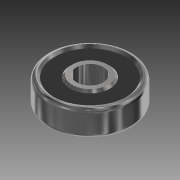
# Autodesk Inventor part: Roulement
Saved by Autodesk Inventor 2016 (Build 200138000, 138)
## iProperties
Created: 2015-04-27
Part Number: Roulement
Material: Générique
Document SubType Name: Modeling
Designer: Logan
Density: 1 g/cm^3
Appearance: Par défaut
Author: Logan
Autodesk Inventor part; units mm, degrees
ref_plane "YZ Plane" through (0, 0, 0) normal (1, 0, 0) x (0, 1, 0)
ref_plane "XZ Plane" through (0, 0, 0) normal (0, 1, 0) x (-1, 0, 0)
ref_plane "XY Plane" through (0, 0, 0) normal (0, 0, 1) x (1, 0, 0)
sketch "Esquisse1" plane through (0, 0, 0) normal (0, 0, 1) x (1, 0, 0)
  circle A0 centre (0, 0) radius 9.5
  circle A1 centre (0, 0) radius 3
  dimension "d0" = 6
  dimension "d1" = 19
  constraints: 2 centre point, 2 coincident
  measures "d0" diameter of A1
  measures "d1" diameter of A0
extrude "Extrusion1" add sketch "Esquisse1" along normal blind 6
fillet "Congé1" radius 1 2 edges at (-9.5, 0, 6) (-9.5, 0, 0)
sketch "Esquisse2" plane through (0, 0, 6) normal (0, 0, 1) x (1, 0, 0)
  circle A0 centre (0, 0) radius 4
  circle A1 centre (0, 0) radius 8.5
  dimension "d5" = 8
  dimension "d6" = 17
  constraints: 2 centre point, 2 coincident
  measures "d5" diameter of A0
  measures "d6" diameter of A1
extrude "Extrusion2" cut sketch "Esquisse2" against normal blind 0.5
sketch "Esquisse3" plane through (0, 0, 0) normal (0, 0, -1) x (-1, 0, 0)
  circle A0 centre (0, 0) radius 4
  circle A1 centre (0, 0) radius 8.5
  constraints: 2 centre point, 2 coincident
extrude "Extrusion3" cut sketch "Esquisse3" against normal blind 0.5
chamfer "Chanfrein3" distance 0.5 angle 45 2 edges at (-4, 0, 5.5) (-8.5, 0, 5.5)
chamfer "Chanfrein4" distance 0.5 angle 45 2 edges at (8.5, 0, 0.5) (4, 0, 0.5)
